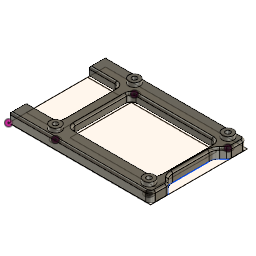
RaspberryPi3B-Sled (Autodesk Fusion 360 design; units mm, degrees)
Autodesk Fusion 360 part; units mm, degrees
sketch "Sketch1" plane through (0, 0, 0) normal (0, 0, 1) x (1, 0, 0) in component "Base"
  line L0 (0, 0) -> (88, 0)
  line L1 (88, 0) -> (88, 60)
  line L2 (88, 60) -> (0, 60)
  line L3 (0, 60) -> (0, 0)
  line L4 (0, 11) -> (20, 11)
  line L5 (20, 11) -> (20, 49)
  line L6 (20, 49) -> (0, 49)
  line L7 (0, 49) -> (0, 11)
  circle A0 centre (23.5, 54.5) radius 1.5
  circle A1 centre (23.5, 5.5) radius 1.5
  circle A2 centre (81.5, 54.5) radius 1.5
  circle A3 centre (81.5, 5.5) radius 1.5
  line L8 (27, 49) -> (80, 49)
  line L9 (80, 49) -> (80, 11)
  line L10 (80, 11) -> (27, 11)
  line L11 (27, 11) -> (27, 49)
  line L12 (88, 48.9236) -> (83, 44)
  line L13 (83, 44) -> (83, 16)
  line L14 (83, 16) -> (88, 10.9224)
  dimension "d3" = 60
  dimension "d4" = 88
  dimension "d14" = 20
  dimension "d15" = 38
  dimension "d16" = 11
  dimension "d18" = 3
  dimension "d19" = 23.5
  dimension "d20" = 3
  dimension "d21" = 23.5
  dimension "d22" = 3
  dimension "d23" = 3
  dimension "d27" = 49
  dimension "d28" = 49
  dimension "d29" = 5.5
  dimension "d30" = 5.5
  dimension "d31" = 7
  dimension "d32" = 8
  dimension "d66" = 58
  dimension "d67" = 58
  dimension "d82" = 38
  dimension "d83" = 11
  measures "d4" distance of L1 L3
  measures "d16" distance of L0 L4
  measures "d18" diameter of A0
  measures "d20" diameter of A1
  measures "d22" diameter of A2
  measures "d23" diameter of A3
  measures "d27" distance of L0.start
  measures "d28" distance of L0.start
  measures "d31" distance of L5 L11
  measures "d32" distance of L1 L9
  measures "d82" distance of L0.start
  measures "d83" distance of L0 L10
extrude "Extrude2" add sketch "Sketch1" along normal blind 6 contours L0 L1 L2 L3 L4 L5 L6 L12 L13 L14 | L1 L12 L13 L14 makes body 1 in component "Base"
extrude "Extrude1" add sketch "Sketch1" along normal blind 6 separate body contours L0 L1 L2 L3 L4 L5 L6 L12 L13 L14 | L1 L12 L13 L14 makes body 2 in component "Base"
sketch "Sketch2" plane through (0, 0, 0) normal (-1, 0, 0) x (0, -1, 0) in component "Base"
  line L0 (-60, 0) -> (-49, 0)
  line L1 (-49, 0) -> (-49, 6)
  line L2 (-49, 6) -> (-60, 6)
  line L3 (-60, 6) -> (-60, 0)
  circle A0 centre (-53.5, 3) radius 1.1
  circle A1 centre (-6.5, 3) radius 1.1
  line L4 (-11, 6) -> (0, 6)
  line L5 (0, 0) -> (0, 6)
  dimension "d35" = 2.2
  dimension "d36" = 2.2
  dimension "d37" = 3
  dimension "d38" = 3
  dimension "d39" = 47
  dimension "d40" = 6.5
  measures "d35" diameter of A0
  measures "d36" diameter of A1
  measures "d37" distance of L2
  measures "d38" distance of L4
  measures "d40" distance of L5
extrude "Extrude3" cut sketch "Sketch2" against normal blind 18 contours A0 | A1 bodies 1 2 in component "Base"
sketch "Sketch3" plane through (0, 0, 6) normal (0, 0, 1) x (-1, 0, 0) in component "Base"
  line L0 (-80, -11) -> (-27, -11)
  line L1 (-27, -11) -> (-27, -49)
  line L2 (-27, -49) -> (-80, -49)
  line L3 (-80, -49) -> (-80, -11)
  circle A0 centre (-81.5, -54.5) radius 1.5
  circle A1 centre (-81.5, -5.5) radius 1.5
  circle A2 centre (-23.5, -5.5) radius 1.5
  circle A3 centre (-23.5, -54.5) radius 1.5
  line L4 (0, -11) -> (0, 0)
  line L5 (0, 0) -> (-88, 0)
  line L6 (-88, 0) -> (-88, -60)
  line L7 (-88, -60) -> (0, -60)
  line L8 (0, -60) -> (0, -49)
  line L9 (0, -49) -> (-20, -49)
  line L10 (-20, -49) -> (-20, -11)
  line L11 (-20, -11) -> (0, -11)
  circle A4 centre (-23.5, -54.5) radius 3.5
  circle A5 centre (-81.5, -54.5) radius 3.5
  circle A6 centre (-81.5, -5.5) radius 3.5
  circle A7 centre (-23.5, -5.5) radius 3.5
  dimension "d43" = 7
  dimension "d45" = 7
  dimension "d46" = 7
  dimension "d47" = 7
  measures "d43" diameter of A4
  measures "d45" diameter of A5
  measures "d46" diameter of A6
  measures "d47" diameter of A7
extrude "Extrude4" add sketch "Sketch3" along normal blind 2.5 contours A4 | A5 | A6 | A7 bodies 1 2 in component "Base"
sketch "Sketch4" plane through (0, 0, 0) normal (0, 0, 1) x (1, 0, 0) in component "Base"
  circle A0 centre (23.5, 5.5) radius 2.75
  circle A1 centre (81.5, 5.5) radius 2.75
  circle A2 centre (81.5, 54.5) radius 2.75
  circle A3 centre (23.5, 54.5) radius 2.75
  dimension "d51" = 5.5
  dimension "d52" = 5.5
  dimension "d53" = 5.5
  dimension "d54" = 5.5
  dimension "d77" = 58
  dimension "d78" = 58
  dimension "d79" = 49
  dimension "d80" = 49
  measures "d51" diameter of A0
  measures "d52" diameter of A1
  measures "d53" diameter of A2
  measures "d54" diameter of A3
  measures "d79" distance of origin
  measures "d80" distance of origin
extrude "Extrude5" cut sketch "Sketch4" along normal blind 4 bodies 1 in component "Base"
fillet "Fillet9" radius 3 12 edges at (80, 49, 3) (80, 49, 3) (20, 49, 3) (20, 49, 3) (80, 11, 3) (80, 11, 3) (20, 11, 3) (20, 11, 3) (27, 49, 3) (27, 49, 3) (27, 11, 3) (27, 11, 3) on bodies 1 2 in component "Base"
chamfer "Chamfer5" distance 1.2 angle 45 13 edges at (27, 30, 0) (27.8787, 48.1213, 0) (53.5, 49, 0) (79.1213, 48.1213, 0) (80, 30, 0) (79.1213, 11.8787, 0) (53.5, 11, 0) (27.8787, 11.8787, 0) (8.5, 11, 0) (19.1213, 11.8787, 0) (20, 30, 0) (19.1213, 48.1213, 0) (8.5, 49, 0) on bodies 1 in component "Base"
fillet "Fillet12" radius 1.2 13 edges at (79.1213, 48.1213, 6) (80, 30, 6) (79.1213, 11.8787, 6) (53.5, 11, 6) (27.8787, 11.8787, 6) (27, 30, 6) (27.8787, 48.1213, 6) (53.5, 49, 6) (8.5, 49, 6) (19.1213, 48.1213, 6) (20, 30, 6) (19.1213, 11.8787, 6) (8.5, 11, 6) on bodies 1 in component "Base"
extrude "Extrude6" cut sketch "Sketch1" along normal up to surface (6 mm away) contours L1 L12 L13 L14 bodies 1 in component "Base"
fillet "Fillet13" radius 6.5 2 edges at (83, 44, 3) (83, 16, 3) on bodies 1 in component "Base"
fillet "Fillet14" radius 3 6 edges at (88, 48.9236, 3) (88, 10.9224, 3) (88, 0, 3) (88, 0, 3) (88, 60, 3) (88, 60, 3) on bodies 1 2 in component "Base"
fillet "Fillet15" radius 1.2 13 edges at (42.5, 0, 6) (87.1213, 0.8787, 6) (88, 6.3466, 6) (87.776, 10.8307, 6) (86.0031, 12.9503, 6) (83.4853, 16.1988, 6) (83, 29.9707, 6) (83.5044, 43.7888, 6) (86.0221, 46.9759, 6) (87.7672, 49.0211, 6) (88, 53.5899, 6) (87.1213, 59.1213, 6) (42.5, 60, 6) on bodies 1 in component "Base"
chamfer "Chamfer8" distance 1 angle 45 14 edges at (0, 49, 3) (0, 49.3515, 5.6485) (0, 54.5, 6) (0, 59.6485, 5.6485) (0, 60, 2.4) (0, 55.1, 0) (0, 49.6, 0.6) (0, 11, 3) (0, 10.6485, 5.6485) (0, 5.5, 6) (0, 0.3515, 5.6485) (0, 0, 2.4) (0, 10.4, 0.6) (0, 4.9, 0) on bodies 1 in component "Base"
component "Base" placed x (1, 0, 0) y (0, 1, 0) z (0, 0, 1) at (0, 0, 0)
equation "width = 82 mm + 6 mm"
equation "height = 60 mm"
equation "d3 = height"
equation "d4 = width"
equation "firstHolesXOffset = 23.5 mm"
equation "secondHolesXOffset = 82 mm"
equation "panelHolesDistance = 47 mm"
equation "piScrewHoleDiameter = 3 mm"
equation "piScrewHeadHoleDiameter = 5.5 mm"
equation "piHoleSpacerDistance = 2.5 mm"
equation "thickness = 6 mm"
equation "d12 = thickness"
equation "d15 = cutoutHeight"
equation "d16 = ( height - cutoutHeight ) / 2"
equation "cutoutHeight = 38 mm"
equation "d18 = piScrewHoleDiameter"
equation "d19 = firstHolesXOffset"
equation "d20 = piScrewHoleDiameter"
equation "d21 = firstHolesXOffset"
equation "d22 = piScrewHoleDiameter"
equation "d23 = piScrewHoleDiameter"
equation "piHolesVerticalSpacing = 49 mm"
equation "d27 = piHolesVerticalSpacing"
equation "d28 = piHolesVerticalSpacing"
equation "d29 = ( height - piHolesVerticalSpacing ) / 2"
equation "d30 = ( height - piHolesVerticalSpacing ) / 2"
equation "d33 = thickness"
equation "d37 = thickness / 2"
equation "d38 = thickness / 2"
equation "d39 = panelHolesDistance"
equation "d40 = ( height - panelHolesDistance ) / 2"
equation "d43 = piSpacerDiameter"
equation "piSpacerDiameter = 7 mm"
equation "d45 = piSpacerDiameter"
equation "d46 = piSpacerDiameter"
equation "d47 = piSpacerDiameter"
equation "d48 = piHoleSpacerDistance"
equation "screwHeadSinkDepth = 4 mm" comment "How far the screw head gets sunk in"
equation "d51 = piScrewHeadHoleDiameter"
equation "d52 = piScrewHeadHoleDiameter"
equation "d53 = piScrewHeadHoleDiameter"
equation "d54 = piScrewHeadHoleDiameter"
equation "d55 = screwHeadSinkDepth"
equation "d82 = cutoutHeight"
equation "d83 = ( height - cutoutHeight ) / 2"
